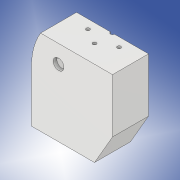
# Autodesk Inventor part: FA002
Saved by Autodesk Inventor 2017 (Build 210142000, 142)
## iProperties
Created: 2017-06-14
Part Number: FA002
Material: ABS Plastic
Document SubType Name: Modeling
Designer: zallen
Density: 1.06 g/cm^3
Appearance: CR White
Author: zallen
Autodesk Inventor part; units mm, degrees
ref_plane "YZ Plane" through (0, 0, 0) normal (1, 0, 0) x (0, 1, 0)
ref_plane "XZ Plane" through (0, 0, 0) normal (0, 1, 0) x (-1, 0, 0)
ref_plane "XY Plane" through (0, 0, 0) normal (0, 0, 1) x (1, 0, 0)
sketch "Sketch1" plane through (0, 0, 0) normal (0, 0, 1) x (1, 0, 0)
  line L0 (0, 0) -> (100, 0)
  line L1 (100, 0) -> (100, -75)
  line L2 (100, -75) -> (75, -118.3013)
  line L3 (75, -118.3013) -> (-12.5, -118.3013)
  line L4 (-12.5, -118.3013) -> (-12.5, -50)
  arc A0 (0, 0) -> (-12.5, -50) centre (77.4072, -45.9143) ccw
  dimension "d0" = 100
  dimension "d1" = 75
  dimension "d2" = 50
  dimension "d3" = 150
  dimension "d5" = 50
  dimension "d6" = 12.5
  dimension "d7" = 90
  constraints: 10 end point, 2 point on circle, 1 centre point, 1 horizontal, 1 parallel, 1 perpendicular, 1 vertical
  measures "d0" distance of L0.start L0.end
  measures "d1" distance of L0.end L1.end
  measures "d2" distance of L1.end L2.end
  measures "d3" angle of L1 L2
  measures "d5" vertical distance of L4.end L0.start
  measures "d6" horizontal distance of L0.start L4.end
  measures "d7" radius of A0
extrude "Extrusion1" add sketch "Sketch1" along normal blind 50
sketch "Sketch2" plane through (0, 0, 0) normal (0, 0, -1) x (-1, 0, 0)
  line L0 (0, 0) -> (-100, 0) projected
  line L1 (-100, 0) -> (-100, -75) projected
  line L2 (-100, -75) -> (-75, -118.3013) projected
  line L3 (-75, -118.3013) -> (12.5, -118.3013) projected
  line L4 (12.5, -118.3013) -> (12.5, -50) projected
  arc A0 (12.5, -50) -> (0, 0) centre (-77.4072, -45.9143) ccw projected
  line L5 (-95, -73.6603) -> (-95, -5)
  line L6 (-95, -5) -> (-2.902, -5)
  arc A1 (7.5, -49.8848) -> (-2.902, -5) centre (-77.4072, -45.9143) ccw
  line L7 (7.5, -49.8848) -> (7.5, -113.3013)
  line L8 (7.5, -113.3013) -> (-72.1132, -113.3013)
  line L9 (-72.1132, -113.3013) -> (-95, -73.6603)
  dimension "d10" = 5
  constraints: 10 end point, 2 point on circle, 1 centre point, 5 other
  measures "d10" distance between parallel lines of L1 L5
extrude "Extrusion2" cut sketch "Sketch2" against normal blind 45 contours L5 L6 A1 L7 L8 L9
sketch "Sketch3" plane through (0, 0, 0) normal (0, 0, -1) x (-1, 0, 0)
  line L0 (7.5, -113.3013) -> (-72.1132, -113.3013) projected
  line L1 (12.5, -118.3013) -> (-75, -118.3013) projected
  line L2 (7.5, -113.3013) -> (-70, -113.3013)
  line L3 (-70, -113.3013) -> (-70, -118.3013)
  line L4 (-70, -118.3013) -> (7.5, -118.3013)
  line L5 (7.5, -118.3013) -> (7.5, -113.3013)
  point P0 (0, 0)
  dimension "d13" = 5
  constraints: 8 end point, 2 parallel, 1 horizontal, 1 perpendicular, 1 point on line
  measures "d13" distance from line of L3 L1.end
extrude "Extrusion3" cut sketch "Sketch3" against normal blind 45
sketch "Sketch4" plane through (0, 0, 0) normal (0, 1, 0) x (1, 0, 0)
  circle A0 centre (50, 0) radius 2.75
  line L0 (0, 0) -> (100, 0) projected
  dimension "d16" = 5.5
  constraints: 1 centre point, 1 coincident, 1 midpoint
  measures "d16" diameter of A0
extrude "Extrusion4" cut sketch "Sketch4" against normal through all
sketch "Sketch5" plane through (0, 0, 50) normal (0, 1, 0) x (1, 0, 0)
  arc A0 (47.25, 50) -> (52.75, 50) centre (50, 50) ccw projected
  circle A1 centre (50, 50) radius 25 construction
  circle A2 centre (50, 25) radius 2.5
  circle A3 centre (71.6506, 37.5) radius 2.5
  circle A4 centre (71.6506, 62.5) radius 2.5
  circle A5 centre (50, 75) radius 2.5
  circle A6 centre (28.3494, 62.5) radius 2.5
  circle A7 centre (28.3494, 37.5) radius 2.5
  point P0 (0, 50)
  dimension "d19" = 50
  dimension "d20" = 5
  dimension "d23" = 360
  constraints: 6 centre point, 2 vertical alignment, 1 coincident, 15 other
  measures "d20" diameter of A2
extrude "Extrusion5" cut sketch "Sketch5" against normal blind 5 contours A2 | A3 | A7
sketch "Sketch6" plane through (0, 0, 50) normal (0, 0, 1) x (1, 0, 0)
  circle A0 centre (25, -25) radius 7.5
  point P0 (0, 0)
  dimension "d27" = 15
  dimension "d28" = 25
  dimension "d29" = 25
  constraints: 1 centre point
  measures "d27" diameter of A0
  measures "d28" horizontal distance of A0.centre point (0, 0)
  measures "d29" horizontal distance of A0.centre point (0, 0)
extrude "Extrusion6" cut sketch "Sketch6" against normal blind 5
body "Solid1"
